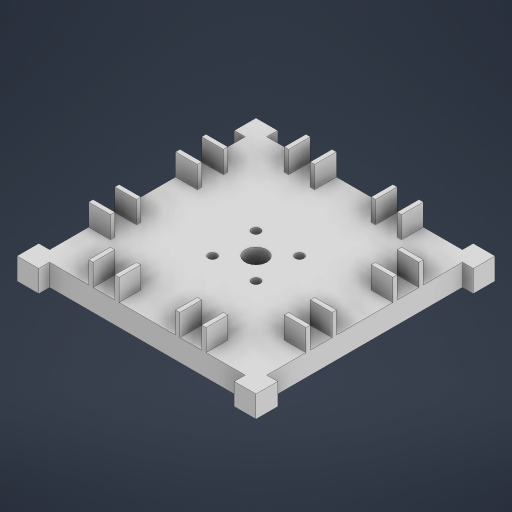
# Autodesk Inventor part: base
Saved by Autodesk Inventor 2024.3 (Build 283343000, 343)
## iProperties
Created: 2024-09-28
Part Number: base
Material: Generic
Document SubType Name: Modeling
Designer: sam
Density: 1 g/cm^3
Appearance: Default
Sheet Metal Rule: Default
Author: sam
Autodesk Inventor part; units mm, degrees
ref_plane "YZ Plane" through (0, 0, 0) normal (1, 0, 0) x (0, 1, 0)
ref_plane "XZ Plane" through (0, 0, 0) normal (0, 1, 0) x (-1, 0, 0)
ref_plane "XY Plane" through (0, 0, 0) normal (0, 0, 1) x (1, 0, 0)
sketch "Sketch1" plane through (0, 0, 0) normal (0, 1, 0) x (-1, 0, 0)
  line L0 (-25, -25) -> (25, -25)
  line L1 (25, -25) -> (25, 25)
  line L2 (25, 25) -> (-25, 25)
  line L3 (-25, 25) -> (-25, -25)
  line L4 (-25, -25) -> (25, 25) construction
  line L5 (25, -25) -> (-25, 25) construction
  circle A0 centre (0, 0) radius 2.5
  line L6 (-22.5, -22.5) -> (-27.5, -22.5)
  line L7 (-27.5, -22.5) -> (-27.5, -27.5)
  line L8 (-27.5, -27.5) -> (-22.5, -27.5)
  line L9 (-22.5, -27.5) -> (-22.5, -22.5)
  line L10 (-22.5, -22.5) -> (-27.5, -27.5) construction
  line L11 (-27.5, -22.5) -> (-22.5, -27.5) construction
  line L12 (27.5, -22.5) -> (22.5, -22.5)
  line L13 (22.5, -22.5) -> (22.5, -27.5)
  line L14 (22.5, -27.5) -> (27.5, -27.5)
  line L15 (27.5, -27.5) -> (27.5, -22.5)
  line L16 (27.5, -22.5) -> (22.5, -27.5) construction
  line L17 (22.5, -22.5) -> (27.5, -27.5) construction
  line L18 (27.5, 27.5) -> (22.5, 27.5)
  line L19 (22.5, 27.5) -> (22.5, 22.5)
  line L20 (22.5, 22.5) -> (27.5, 22.5)
  line L21 (27.5, 22.5) -> (27.5, 27.5)
  line L22 (27.5, 27.5) -> (22.5, 22.5) construction
  line L23 (22.5, 27.5) -> (27.5, 22.5) construction
  line L24 (-22.5, 27.5) -> (-27.5, 27.5)
  line L25 (-27.5, 27.5) -> (-27.5, 22.5)
  line L26 (-27.5, 22.5) -> (-22.5, 22.5)
  line L27 (-22.5, 22.5) -> (-22.5, 27.5)
  line L28 (-22.5, 27.5) -> (-27.5, 22.5) construction
  line L29 (-27.5, 27.5) -> (-22.5, 22.5) construction
  circle A1 centre (5, -5) radius 1
  circle A2 centre (5, 5) radius 1
  circle A3 centre (-5, 5) radius 1
  circle A4 centre (-5, -5) radius 1
  point P0 (25, -22.5)
  point P1 (22.5, -25)
  point P2 (-22.5, -25)
  point P3 (-25, -22.5)
  point P4 (-25, 22.5)
  point P5 (-22.5, 25)
  point P6 (22.5, 25)
  point P7 (25, 22.5)
  point P8 (0, -25)
  point P9 (25, 0)
  point P10 (0, 25)
  point P11 (-25, 0)
  dimension "d0" = 50
  dimension "d1" = 50
  dimension "d45" = 5
  dimension "d46" = 5
  dimension "d47" = 5
  dimension "d48" = 5
  dimension "d49" = 5
  dimension "d50" = 5
  dimension "d51" = 5
  dimension "d52" = 5
  dimension "d53" = 5
  dimension "d82" = 2
  dimension "d83" = 2
  dimension "d84" = 2
  dimension "d85" = 2
  dimension "d86" = 5
  dimension "d87" = 5
  dimension "d88" = 5
  dimension "d89" = 5
  dimension "d90" = 5
  dimension "d91" = 5
  dimension "d92" = 5
  dimension "d93" = 5
  constraints: 60 end point, 14 midpoint, 10 parallel, 5 centre point, 5 horizontal, 5 perpendicular, 1 coincident
  measures "d0" distance of L2.end L1.end
  measures "d1" distance of L1.end L0.end
  measures "d45" diameter of A0
  measures "d46" distance of L8.end L7.end
  measures "d47" distance of L7.end L6.end
  measures "d48" distance of L14.end L13.end
  measures "d49" distance of L13.end L12.end
  measures "d50" distance of L20.end L19.end
  measures "d51" distance of L19.end L18.end
  measures "d52" distance of L26.end L25.end
  measures "d53" distance of L25.end L24.end
  measures "d82" diameter of A1
  measures "d83" diameter of A2
  measures "d84" diameter of A3
  measures "d85" diameter of A4
  measures "d86" horizontal distance of point (0, -25) A4.centre
  measures "d87" horizontal distance of A1.centre point (0, -25)
  measures "d88" vertical distance of point (25, 0) A1.centre
  measures "d89" vertical distance of point (25, 0) A2.centre
  measures "d90" horizontal distance of point (0, 25) A2.centre
  measures "d91" horizontal distance of point (0, 25) A3.centre
  measures "d92" vertical distance of point (-25, 0) A3.centre
  measures "d93" vertical distance of point (-25, 0) A4.centre
extrude "Extrusion1" add sketch "Sketch1" along normal blind 5
sketch "Sketch2" plane through (0, 5, 0) normal (0, 1, 0) x (1, 0, 0)
  line L0 (-25, 22.5) -> (-25, -22.5) projected
  line L1 (-22.5, -25) -> (22.5, -25) projected
  line L2 (25, -22.5) -> (25, 22.5) projected
  line L3 (22.5, 25) -> (-22.5, 25) projected
  line L4 (25, -12.5) -> (20, -12.5)
  line L5 (20, -12.5) -> (20, -7.5)
  line L6 (20, -7.5) -> (25, -7.5)
  line L7 (25, -7.5) -> (25, -12.5)
  line L8 (25, -22.5) -> (25, 22.5) projected
  line L9 (25, 7.5) -> (20, 7.5)
  line L10 (20, 7.5) -> (20, 12.5)
  line L11 (20, 12.5) -> (25, 12.5)
  line L12 (25, 12.5) -> (25, 7.5)
  line L13 (-25, -12.5) -> (-20, -12.5)
  line L14 (-20, -12.5) -> (-20, -7.5)
  line L15 (-20, -7.5) -> (-25, -7.5)
  line L16 (-25, -7.5) -> (-25, -12.5)
  line L17 (-25, 22.5) -> (-25, -22.5) projected
  line L18 (-25, 7.5) -> (-20, 7.5)
  line L19 (-20, 7.5) -> (-20, 12.5)
  line L20 (-20, 12.5) -> (-25, 12.5)
  line L21 (-25, 12.5) -> (-25, 7.5)
  line L22 (-22.5, -25) -> (22.5, -25) projected
  line L23 (-25, 12.5) -> (-20, 12.5)
  line L24 (-20, 12.5) -> (-20, 13.5)
  line L25 (-20, 13.5) -> (-25, 13.5)
  line L26 (-25, 13.5) -> (-25, 12.5)
  line L27 (20, 12.5) -> (25, 12.5)
  line L28 (25, 12.5) -> (25, 13.5)
  line L29 (25, 13.5) -> (20, 13.5)
  line L30 (20, 13.5) -> (20, 12.5)
  line L31 (25, 7.5) -> (20, 7.5)
  line L32 (20, 7.5) -> (20, 6.5)
  line L33 (20, 6.5) -> (25, 6.5)
  line L34 (25, 6.5) -> (25, 7.5)
  line L35 (-20, 7.5) -> (-25, 7.5)
  line L36 (-25, 7.5) -> (-25, 6.5)
  line L37 (-25, 6.5) -> (-20, 6.5)
  line L38 (-20, 6.5) -> (-20, 7.5)
  line L39 (-25, -7.5) -> (-20, -7.5)
  line L40 (-20, -7.5) -> (-20, -6.5)
  line L41 (-20, -6.5) -> (-25, -6.5)
  line L42 (-25, -6.5) -> (-25, -7.5)
  line L43 (-25, -12.5) -> (-20, -12.5)
  line L44 (-20, -12.5) -> (-20, -13.5)
  line L45 (-20, -13.5) -> (-25, -13.5)
  line L46 (-25, -13.5) -> (-25, -12.5)
  line L47 (25, -7.5) -> (20, -7.5)
  line L48 (20, -7.5) -> (20, -6.5)
  line L49 (20, -6.5) -> (25, -6.5)
  line L50 (25, -6.5) -> (25, -7.5)
  line L51 (20, -12.5) -> (25, -12.5)
  line L52 (25, -12.5) -> (25, -13.5)
  line L53 (25, -13.5) -> (20, -13.5)
  line L54 (20, -13.5) -> (20, -12.5)
  line L55 (-25, -22.5) -> (-27.5, -22.5) projected
  line L56 (-27.5, -22.5) -> (-27.5, -27.5) projected
  line L57 (-27.5, -27.5) -> (-22.5, -27.5) projected
  line L58 (-22.5, -27.5) -> (-22.5, -25) projected
  line L59 (22.5, -25) -> (22.5, -27.5) projected
  line L60 (22.5, -27.5) -> (27.5, -27.5) projected
  line L61 (27.5, -27.5) -> (27.5, -22.5) projected
  line L62 (27.5, -22.5) -> (25, -22.5) projected
  line L63 (25, 22.5) -> (27.5, 22.5) projected
  line L64 (27.5, 22.5) -> (27.5, 27.5) projected
  line L65 (27.5, 27.5) -> (22.5, 27.5) projected
  line L66 (22.5, 27.5) -> (22.5, 25) projected
  line L67 (-22.5, 25) -> (-22.5, 27.5) projected
  line L68 (-22.5, 27.5) -> (-27.5, 27.5) projected
  line L69 (-27.5, 27.5) -> (-27.5, 22.5) projected
  line L70 (-27.5, 22.5) -> (-25, 22.5) projected
  line L71 (-12.5, 25) -> (-7.5, 25)
  line L72 (-7.5, 25) -> (-7.5, 20)
  line L73 (-7.5, 20) -> (-12.5, 20)
  line L74 (-12.5, 20) -> (-12.5, 25)
  line L75 (7.5, 25) -> (12.5, 25)
  line L76 (12.5, 25) -> (12.5, 20)
  line L77 (12.5, 20) -> (7.5, 20)
  line L78 (7.5, 20) -> (7.5, 25)
  line L79 (-12.5, -25) -> (-7.5, -25)
  line L80 (-7.5, -25) -> (-7.5, -20)
  line L81 (-7.5, -20) -> (-12.5, -20)
  line L82 (-12.5, -20) -> (-12.5, -25)
  line L83 (7.5, -25) -> (12.5, -25)
  line L84 (12.5, -25) -> (12.5, -20)
  line L85 (12.5, -20) -> (7.5, -20)
  line L86 (7.5, -20) -> (7.5, -25)
  line L87 (22.5, 25) -> (-22.5, 25) projected
  line L88 (-12.5, -20) -> (-13.5, -20)
  line L89 (-13.5, -20) -> (-13.5, -25)
  line L90 (-13.5, -25) -> (-12.5, -25)
  line L91 (-12.5, -25) -> (-12.5, -20)
  line L92 (-7.5, -20) -> (-6.5, -20)
  line L93 (-6.5, -20) -> (-6.5, -25)
  line L94 (-6.5, -25) -> (-7.5, -25)
  line L95 (-7.5, -25) -> (-7.5, -20)
  line L96 (7.5, -20) -> (6.5, -20)
  line L97 (6.5, -20) -> (6.5, -25)
  line L98 (6.5, -25) -> (7.5, -25)
  line L99 (7.5, -25) -> (7.5, -20)
  line L100 (12.5, -20) -> (13.5, -20)
  line L101 (13.5, -20) -> (13.5, -25)
  line L102 (13.5, -25) -> (12.5, -25)
  line L103 (12.5, -25) -> (12.5, -20)
  line L104 (-7.5, 25) -> (-6.5, 25)
  line L105 (-6.5, 25) -> (-6.5, 20)
  line L106 (-6.5, 20) -> (-7.5, 20)
  line L107 (-7.5, 20) -> (-7.5, 25)
  line L108 (7.5, 25) -> (6.5, 25)
  line L109 (6.5, 25) -> (6.5, 20)
  line L110 (6.5, 20) -> (7.5, 20)
  line L111 (7.5, 20) -> (7.5, 25)
  line L112 (12.5, 25) -> (13.5, 25)
  line L113 (13.5, 25) -> (13.5, 20)
  line L114 (13.5, 20) -> (12.5, 20)
  line L115 (12.5, 20) -> (12.5, 25)
  line L116 (-12.5, 25) -> (-13.5, 25)
  line L117 (-13.5, 25) -> (-13.5, 20)
  line L118 (-13.5, 20) -> (-12.5, 20)
  line L119 (-12.5, 20) -> (-12.5, 25)
  point P0 (0, 0)
  point P1 (-25, 25)
  point P2 (-25, -25)
  point P3 (25, -25)
  point P4 (25, 25)
  point P5 (20, -10)
  point P6 (20, 10)
  point P7 (-25, 10)
  point P8 (-25, -10)
  point P9 (-25, 6.5)
  point P10 (-25, 13.5)
  point P11 (25, 13.5)
  point P12 (25, 6.5)
  point P13 (25, -13.5)
  point P14 (-25, -13.5)
  point P15 (25, 10)
  point P16 (-25, 0)
  point P17 (0, -25)
  point P18 (-10, -25)
  point P19 (10, -25)
  point P20 (0, 25)
  point P21 (10, 25)
  point P22 (-10, 25)
  point P23 (0, 25)
  dimension "d9" = 5
  dimension "d10" = 5
  dimension "d11" = 5
  dimension "d12" = 5
  dimension "d13" = 5
  dimension "d14" = 5
  dimension "d15" = 5
  dimension "d16" = 5
  dimension "d21" = 5
  dimension "d22" = 1
  dimension "d23" = 5
  dimension "d24" = 1
  dimension "d25" = 5
  dimension "d26" = 1
  dimension "d27" = 5
  dimension "d28" = 1
  dimension "d29" = 5
  dimension "d30" = 1
  dimension "d31" = 5
  dimension "d32" = 1
  dimension "d33" = 5
  dimension "d34" = 1
  dimension "d35" = 5
  dimension "d36" = 1
  dimension "d43" = 10
  dimension "d54" = 5
  dimension "d55" = 5
  dimension "d56" = 5
  dimension "d57" = 5
  dimension "d58" = 5
  dimension "d59" = 5
  dimension "d60" = 5
  dimension "d61" = 5
  dimension "d62" = 10
  dimension "d63" = 10
  dimension "d64" = 10
  dimension "d65" = 10
  dimension "d66" = 1
  dimension "d67" = 5
  dimension "d68" = 1
  dimension "d69" = 5
  dimension "d70" = 1
  dimension "d71" = 5
  dimension "d72" = 1
  dimension "d73" = 5
  dimension "d74" = 1
  dimension "d75" = 5
  dimension "d76" = 1
  dimension "d77" = 5
  dimension "d78" = 1
  dimension "d79" = 5
  dimension "d80" = 1
  dimension "d81" = 5
  constraints: 192 end point, 48 parallel, 24 horizontal, 24 perpendicular, 12 midpoint, 8 point on line, 2 other
  measures "d9" distance of L5.end L6.end
  measures "d10" distance of L4.end L5.end
  measures "d11" distance of L10.end L11.end
  measures "d12" distance of L9.end L10.end
  measures "d13" distance of L15.end L14.end
  measures "d14" distance of L14.end L13.end
  measures "d15" distance of L20.end L19.end
  measures "d16" distance of L19.end L18.end
  measures "d21" distance of L25.end L24.end
  measures "d22" distance of L24.end L23.end
  measures "d23" distance of L29.end L28.end
  measures "d24" distance of L28.end L27.end
  measures "d25" distance of L33.end L32.end
  measures "d26" distance of L32.end L31.end
  measures "d27" distance of L37.end L36.end
  measures "d28" distance of L36.end L35.end
  measures "d29" distance of L41.end L40.end
  measures "d30" distance of L40.end L39.end
  measures "d31" distance of L44.end L45.end
  measures "d32" distance of L43.end L44.end
  measures "d33" distance of L48.end L49.end
  measures "d34" distance of L47.end L48.end
  measures "d35" distance of L52.end L53.end
  measures "d36" distance of L51.end L52.end
  measures "d43" distance of point (-25, 0) point (-25, 10)
  measures "d54" distance of L72.end L73.end
  measures "d55" distance of L71.end L72.end
  measures "d56" distance of L76.end L77.end
  measures "d57" distance of L75.end L76.end
  measures "d58" distance of L81.end L80.end
  measures "d59" distance between parallel lines of L81 L1
  measures "d60" distance of L85.end L84.end
  measures "d61" distance of L84.end L83.end
  measures "d62" distance of point (0, -25) point (-10, -25)
  measures "d63" distance of point (10, -25) point (0, -25)
  measures "d64" distance of point (0, 25) point (10, 25)
  measures "d65" distance of point (-10, 25) point (0, 25)
  measures "d66" distance of L90.end L89.end
  measures "d67" distance of L89.end L88.end
  measures "d68" distance of L93.end L94.end
  measures "d69" distance of L92.end L93.end
  measures "d70" distance of L98.end L97.end
  measures "d71" distance of L97.end L96.end
  measures "d72" distance of L101.end L102.end
  measures "d73" distance of L100.end L101.end
  measures "d74" distance of L105.end L106.end
  measures "d75" distance of L104.end L105.end
  measures "d76" distance of L110.end L109.end
  measures "d77" distance of L109.end L108.end
  measures "d78" distance of L113.end L114.end
  measures "d79" distance of L112.end L113.end
  measures "d80" distance of L118.end L117.end
  measures "d81" distance of L117.end L116.end
extrude "Extrusion2" add sketch "Sketch2" along normal blind 5 contours L25 L24 L20 L0 | L18 L38 L37 L0 | L41 L40 L15 L0 | L3 L74 L118 L117 | L13 L44 L45 L0 | L3 L105 L106 L72 | L3 L78 L110 L109 | L3 L113 L114 L76 | L89 L88 L82 L1 | L80 L92 L93 L1 | L97 L96 L86 L1 | L2 L11 L30 L29 | L84 L100 L101 L1 | L2 L33 L32 L9 | L2 L6 L48 L49 | L2 L53 L54 L4
equation "\"BendRadius\" = Thickness"
equation "\"BendReliefWidth\" = Thickness"
equation "\"BendReliefDepth\" = 0.5 * Thickness"
equation "\"CornerReliefSize\" = 4 * Thickness"
equation "\"MinimumRemnant\" = 2 * Thickness"
equation "\"TransitionRadius\" = BendRadius"
equation "\"JacobiRadiusSize\" = BendRadius"
equation "\"GapSize\" = Thickness"
equation "\"Thickness\" = 3.048"
body "Solid1"
